Autodesk Inventor part; units mm, degrees
(part 2 of 2)
sketch "Sketch2" plane through (-23.7091, -13.8536, 14.2492) normal (0, 0.9970894, 0.0762418) x (1, 0, 0)
  line L0 (0.0409, 0.625) -> (-23.5591, 0.625) projected
  line L1 (0.0409, 0.625) -> (-23.5591, 0.625)
  line L2 (-23.5591, 0.625) -> (-23.5591, 65.9208)
  line L3 (-23.5591, 65.9208) -> (0.0409, 65.9208)
  line L4 (0.0409, 65.9208) -> (0.0409, 0.625)
  circle A0 centre (-9.1675, 23.6102) radius 8 construction
  circle A1 centre (-12.9591, 35.6262) radius 9.6 construction
  circle A2 centre (-9.1675, 23.6102) radius 8.4
  circle A3 centre (-12.9591, 35.6262) radius 10
  circle A4 centre (-9.1675, 23.6102) radius 1.25 projected
  arc A5 (-17.1384, 22.9282) -> (-15.9774, 22.6664) centre (-15.4653, 27.6426) ccw projected
  arc A6 (-15.9774, 22.6664) -> (-15.9187, 22.3113) centre (-9.1675, 23.6102) ccw projected
  arc A7 (-15.9187, 22.3113) -> (-16.9336, 21.6897) centre (-13.8318, 17.7649) ccw projected
  arc A8 (-16.9336, 21.6897) -> (-16.8224, 21.2858) centre (-9.1675, 23.6102) ccw projected
  arc A9 (-16.8224, 21.2858) -> (-15.6324, 21.2712) centre (-16.1661, 26.2451) ccw projected
  arc A10 (-15.6324, 21.2712) -> (-15.5011, 20.936) centre (-9.1675, 23.6102) ccw projected
  arc A11 (-15.5011, 20.936) -> (-16.3646, 20.117) centre (-12.5145, 16.9228) ccw projected
  arc A12 (-16.3646, 20.117) -> (-16.1719, 19.7451) centre (-9.1675, 23.6102) ccw projected
  arc A13 (-16.1719, 19.7451) -> (-15.0048, 19.9781) centre (-16.561, 24.7325) ccw projected
  arc A14 (-15.0048, 19.9781) -> (-14.8067, 19.6776) centre (-9.1675, 23.6102) ccw projected
  arc A15 (-14.8067, 19.6776) -> (-15.481, 18.697) centre (-11.051, 16.3731) ccw projected
  arc A16 (-15.481, 18.697) -> (-15.2152, 18.3733) centre (-9.1675, 23.6102) ccw projected
  arc A17 (-15.2152, 18.3733) -> (-14.1221, 18.8439) centre (-16.6328, 23.1708) ccw projected
  arc A18 (-14.1221, 18.8439) -> (-13.8659, 18.5911) centre (-9.1675, 23.6102) ccw projected
  arc A19 (-13.8659, 18.5911) -> (-14.3215, 17.4917) centre (-9.5052, 16.1397) ccw projected
  arc A20 (-14.3215, 17.4917) -> (-13.9942, 17.2303) centre (-9.1675, 23.6102) ccw projected
  arc A21 (-13.9942, 17.2303) -> (-13.0229, 17.9179) centre (-16.3783, 21.6283) ccw projected
  arc A22 (-13.0229, 17.9179) -> (-12.7197, 17.7239) centre (-9.1675, 23.6102) ccw projected
  arc A23 (-12.7197, 17.7239) -> (-12.9368, 16.5538) centre (-7.9446, 16.2327) ccw projected
  arc A24 (-12.9368, 16.5538) -> (-12.5623, 16.3662) centre (-9.1675, 23.6102) ccw projected
  arc A25 (-12.5623, 16.3662) -> (-11.7551, 17.2407) centre (-15.8086, 20.1724) ccw projected
  arc A26 (-11.7551, 17.2407) -> (-11.4182, 17.114) centre (-9.1675, 23.6102) ccw projected
  arc A27 (-11.4182, 17.114) -> (-11.3873, 15.9243) centre (-6.4374, 16.6482) ccw projected
  arc A28 (-11.3873, 15.9243) -> (-10.982, 15.8187) centre (-9.1675, 23.6102) ccw projected
  arc A29 (-10.982, 15.8187) -> (-10.3743, 16.8419) centre (-14.9487, 18.8667) ccw projected
  arc A30 (-10.3743, 16.8419) -> (-10.0184, 16.7881) centre (-9.1675, 23.6102) ccw projected
  arc A31 (-10.0184, 16.7881) -> (-9.7408, 15.6308) centre (-5.0496, 17.3679) ccw projected
  arc A32 (-9.7408, 15.6308) -> (-9.3224, 15.6117) centre (-9.1675, 23.6102) ccw projected
  arc A33 (-9.3224, 15.6117) -> (-8.9407, 16.7389) centre (-13.8362, 17.7684) ccw projected
  arc A34 (-8.9407, 16.7389) -> (-8.5814, 16.7602) centre (-9.1675, 23.6102) ccw projected
  arc A35 (-8.5814, 16.7602) -> (-8.0693, 15.6859) centre (-3.8418, 18.3605) ccw projected
  arc A36 (-8.0693, 15.6859) -> (-7.6561, 15.7543) centre (-9.1675, 23.6102) ccw projected
  arc A37 (-7.6561, 15.7543) -> (-7.5171, 16.9362) centre (-12.5196, 16.9254) ccw projected
  arc A38 (-7.5171, 16.9362) -> (-7.17, 17.0318) centre (-9.1675, 23.6102) ccw projected
  arc A39 (-7.17, 17.0318) -> (-6.4457, 16.0874) centre (-2.8667, 19.5825) ccw projected
  arc A40 (-6.4457, 16.0874) -> (-6.0558, 16.2402) centre (-9.1675, 23.6102) ccw projected
  arc A41 (-6.0558, 16.2402) -> (-6.1655, 17.4252) centre (-11.0565, 16.3745) ccw projected
  arc A42 (-6.1655, 17.4252) -> (-5.846, 17.5908) centre (-9.1675, 23.6102) ccw projected
  arc A43 (-5.846, 17.5908) -> (-4.9411, 16.8177) centre (-2.167, 20.9806) ccw projected
  arc A44 (-4.9411, 16.8177) -> (-4.5914, 17.0482) centre (-9.1675, 23.6102) ccw projected
  arc A45 (-4.5914, 17.0482) -> (-4.9452, 18.1845) centre (-9.5108, 16.1399) ccw projected
  arc A46 (-4.9452, 18.1845) -> (-4.667, 18.413) centre (-9.1675, 23.6102) ccw projected
  arc A47 (-4.667, 18.413) -> (-3.6213, 17.8449) centre (-1.7732, 22.4935) ccw projected
  arc A48 (-3.6213, 17.8449) -> (-3.3271, 18.143) centre (-9.1675, 23.6102) ccw projected
  arc A49 (-3.3271, 18.143) -> (-3.9094, 19.181) centre (-7.9502, 16.2318) ccw projected
  arc A50 (-3.9094, 19.181) -> (-3.6848, 19.4622) centre (-9.1675, 23.6102) ccw projected
  arc A51 (-3.6848, 19.4622) -> (-2.5438, 19.124) centre (-1.7026, 24.0553) ccw projected
  arc A52 (-2.5438, 19.124) -> (-2.3181, 19.4768) centre (-9.1675, 23.6102) ccw projected
  arc A53 (-2.3181, 19.4768) -> (-3.1034, 20.371) centre (-6.4427, 16.6461) ccw projected
  arc A54 (-3.1034, 20.371) -> (-2.9422, 20.6928) centre (-9.1675, 23.6102) ccw projected
  arc A55 (-2.9422, 20.6928) -> (-1.7558, 20.5992) centre (-1.9583, 25.5976) ccw projected
  arc A56 (-1.7558, 20.5992) -> (-1.6084, 20.9912) centre (-9.1675, 23.6102) ccw projected
  arc A57 (-1.6084, 20.9912) -> (-2.5625, 21.7026) centre (-5.0543, 17.3648) ccw projected
  arc A58 (-2.5625, 21.7026) -> (-2.4717, 22.0509) centre (-9.1675, 23.6102) ccw projected
  arc A59 (-2.4717, 22.0509) -> (-1.2917, 22.206) centre (-2.529, 27.0531) ccw projected
  arc A60 (-1.2917, 22.206) -> (-1.229, 22.6201) centre (-9.1675, 23.6102) ccw projected
  arc A61 (-1.229, 22.6201) -> (-2.3102, 23.1175) centre (-3.8457, 18.3565) ccw projected
  arc A62 (-2.3102, 23.1175) -> (-2.2938, 23.4771) centre (-9.1675, 23.6102) ccw projected
  arc A63 (-2.2938, 23.4771) -> (-1.1719, 23.8741) centre (-3.3899, 28.3581) ccw projected
  arc A64 (-1.1719, 23.8741) -> (-1.1967, 24.2922) centre (-9.1675, 23.6102) ccw projected
  arc A65 (-1.1967, 24.2922) -> (-2.3576, 24.554) centre (-2.8697, 19.5777) ccw projected
  arc A66 (-2.3576, 24.554) -> (-2.4163, 24.9091) centre (-9.1675, 23.6102) ccw projected
  arc A67 (-2.4163, 24.9091) -> (-1.4015, 25.5307) centre (-4.5033, 29.4555) ccw projected
  arc A68 (-1.4015, 25.5307) -> (-1.5126, 25.9345) centre (-9.1675, 23.6102) ccw projected
  arc A69 (-1.5126, 25.9345) -> (-2.7027, 25.9492) centre (-2.169, 20.9752) ccw projected
  arc A70 (-2.7027, 25.9492) -> (-2.8339, 26.2844) centre (-9.1675, 23.6102) ccw projected
  arc A71 (-2.8339, 26.2844) -> (-1.9705, 27.1034) centre (-5.8205, 30.2975) ccw projected
  arc A72 (-1.9705, 27.1034) -> (-2.1632, 27.4753) centre (-9.1675, 23.6102) ccw projected
  arc A73 (-2.1632, 27.4753) -> (-3.3302, 27.2422) centre (-1.7741, 22.4879) ccw projected
  arc A74 (-3.3302, 27.2422) -> (-3.5283, 27.5428) centre (-9.1675, 23.6102) ccw projected
  arc A75 (-3.5283, 27.5428) -> (-2.854, 28.5234) centre (-7.2841, 30.8473) ccw projected
  arc A76 (-2.854, 28.5234) -> (-3.1198, 28.8471) centre (-9.1675, 23.6102) ccw projected
  arc A77 (-3.1198, 28.8471) -> (-4.213, 28.3765) centre (-1.7023, 24.0496) ccw projected
  arc A78 (-4.213, 28.3765) -> (-4.4692, 28.6293) centre (-9.1675, 23.6102) ccw projected
  arc A79 (-4.4692, 28.6293) -> (-4.0135, 29.7287) centre (-8.8299, 31.0807) ccw projected
  arc A80 (-4.0135, 29.7287) -> (-4.3408, 29.9901) centre (-9.1675, 23.6102) ccw projected
  arc A81 (-4.3408, 29.9901) -> (-5.3122, 29.3025) centre (-1.9568, 25.5921) ccw projected
  arc A82 (-5.3122, 29.3025) -> (-5.6154, 29.4964) centre (-9.1675, 23.6102) ccw projected
  arc A83 (-5.6154, 29.4964) -> (-5.3983, 30.6666) centre (-10.3905, 30.9877) ccw projected
  arc A84 (-5.3983, 30.6666) -> (-5.7727, 30.8542) centre (-9.1675, 23.6102) ccw projected
  arc A85 (-5.7727, 30.8542) -> (-6.5799, 29.9797) centre (-2.5264, 27.048) ccw projected
  arc A86 (-6.5799, 29.9797) -> (-6.9168, 30.1063) centre (-9.1675, 23.6102) ccw projected
  arc A87 (-6.9168, 30.1063) -> (-6.9477, 31.2961) centre (-11.8976, 30.5722) ccw projected
  arc A88 (-6.9477, 31.2961) -> (-7.353, 31.4017) centre (-9.1675, 23.6102) ccw projected
  arc A89 (-7.353, 31.4017) -> (-7.9608, 30.3785) centre (-3.3863, 28.3537) ccw projected
  arc A90 (-7.9608, 30.3785) -> (-8.3166, 30.4323) centre (-9.1675, 23.6102) ccw projected
  arc A91 (-8.3166, 30.4323) -> (-8.5942, 31.5896) centre (-13.2855, 29.8524) ccw projected
  arc A92 (-8.5942, 31.5896) -> (-9.0126, 31.6087) centre (-9.1675, 23.6102) ccw projected
  arc A93 (-9.0126, 31.6087) -> (-9.3943, 30.4815) centre (-4.4989, 29.452) ccw projected
  arc A94 (-9.3943, 30.4815) -> (-9.7536, 30.4602) centre (-9.1675, 23.6102) ccw projected
  arc A95 (-9.7536, 30.4602) -> (-10.2658, 31.5345) centre (-14.4933, 28.8599) ccw projected
  arc A96 (-10.2658, 31.5345) -> (-10.679, 31.4661) centre (-9.1675, 23.6102) ccw projected
  arc A97 (-10.679, 31.4661) -> (-10.818, 30.2841) centre (-5.8155, 30.295) ccw projected
  arc A98 (-10.818, 30.2841) -> (-11.165, 30.1886) centre (-9.1675, 23.6102) ccw projected
  arc A99 (-11.165, 30.1886) -> (-11.8893, 31.1329) centre (-15.4684, 27.6379) ccw projected
  arc A100 (-11.8893, 31.1329) -> (-12.2793, 30.9802) centre (-9.1675, 23.6102) ccw projected
  arc A101 (-12.2793, 30.9802) -> (-12.1695, 29.7952) centre (-7.2786, 30.8459) ccw projected
  arc A102 (-12.1695, 29.7952) -> (-12.4891, 29.6296) centre (-9.1675, 23.6102) ccw projected
  arc A103 (-12.4891, 29.6296) -> (-13.3939, 30.4027) centre (-16.1681, 26.2398) ccw projected
  arc A104 (-13.3939, 30.4027) -> (-13.7436, 30.1722) centre (-9.1675, 23.6102) ccw projected
  arc A105 (-13.7436, 30.1722) -> (-13.3898, 29.0358) centre (-8.8242, 31.0805) ccw projected
  arc A106 (-13.3898, 29.0358) -> (-13.668, 28.8074) centre (-9.1675, 23.6102) ccw projected
  arc A107 (-13.668, 28.8074) -> (-14.7138, 29.3755) centre (-16.5619, 24.7269) ccw projected
  arc A108 (-14.7138, 29.3755) -> (-15.0079, 29.0774) centre (-9.1675, 23.6102) ccw projected
  arc A109 (-15.0079, 29.0774) -> (-14.4256, 28.0394) centre (-10.3849, 30.9886) ccw projected
  arc A110 (-14.4256, 28.0394) -> (-14.6502, 27.7582) centre (-9.1675, 23.6102) ccw projected
  arc A111 (-14.6502, 27.7582) -> (-15.7913, 28.0964) centre (-16.6324, 23.1651) ccw projected
  arc A112 (-15.7913, 28.0964) -> (-16.017, 27.7436) centre (-9.1675, 23.6102) ccw projected
  arc A113 (-16.017, 27.7436) -> (-15.2316, 26.8494) centre (-11.8923, 30.5743) ccw projected
  arc A114 (-15.2316, 26.8494) -> (-15.3928, 26.5276) centre (-9.1675, 23.6102) ccw projected
  arc A115 (-15.3928, 26.5276) -> (-16.5793, 26.6212) centre (-16.3768, 21.6228) ccw projected
  arc A116 (-16.5793, 26.6212) -> (-16.7267, 26.2292) centre (-9.1675, 23.6102) ccw projected
  arc A117 (-16.7267, 26.2292) -> (-15.7726, 25.5178) centre (-13.2807, 29.8556) ccw projected
  arc A118 (-15.7726, 25.5178) -> (-15.8634, 25.1695) centre (-9.1675, 23.6102) ccw projected
  arc A119 (-15.8634, 25.1695) -> (-17.0433, 25.0144) centre (-15.806, 20.1673) ccw projected
  arc A120 (-17.0433, 25.0144) -> (-17.106, 24.6003) centre (-9.1675, 23.6102) ccw projected
  arc A121 (-17.106, 24.6003) -> (-16.0249, 24.1029) centre (-14.4893, 28.8639) ccw projected
  arc A122 (-16.0249, 24.1029) -> (-16.0412, 23.7433) centre (-9.1675, 23.6102) ccw projected
  arc A123 (-16.0412, 23.7433) -> (-17.1632, 23.3463) centre (-14.9451, 18.8623) ccw projected
  arc A124 (-17.1632, 23.3463) -> (-17.1384, 22.9282) centre (-9.1675, 23.6102) ccw projected
  arc A125 (-20.5914, 38.7585) -> (-22.0189, 38.8013) centre (-21.4836, 32.8221) ccw projected
  arc A126 (-22.0189, 38.8013) -> (-22.1726, 38.3228) centre (-12.9591, 35.6262) ccw projected
  arc A127 (-22.1726, 38.3228) -> (-20.9874, 37.526) centre (-18.2546, 42.8709) ccw projected
  arc A128 (-20.9874, 37.526) -> (-21.0758, 37.1032) centre (-12.9591, 35.6262) ccw projected
  arc A129 (-21.0758, 37.1032) -> (-22.481, 36.8482) centre (-20.7143, 31.1111) ccw projected
  arc A130 (-22.481, 36.8482) -> (-22.5319, 36.3482) centre (-12.9591, 35.6262) ccw projected
  arc A131 (-22.5319, 36.3482) -> (-21.207, 35.8153) centre (-19.6452, 41.6116) ccw projected
  arc A132 (-21.207, 35.8153) -> (-21.2056, 35.3834) centre (-12.9591, 35.6262) ccw projected
  arc A133 (-21.2056, 35.3834) -> (-22.527, 34.8418) centre (-19.6061, 29.5973) ccw projected
  arc A134 (-22.527, 34.8418) -> (-22.4729, 34.3422) centre (-12.9591, 35.6262) ccw projected
  arc A135 (-22.4729, 34.3422) -> (-21.066, 34.0963) centre (-20.7435, 40.0907) ccw projected
  arc A136 (-21.066, 34.0963) -> (-20.9749, 33.6742) centre (-12.9591, 35.6262) ccw projected
  arc A137 (-20.9749, 33.6742) -> (-22.1549, 32.8697) centre (-18.2074, 28.3471) ccw projected
  arc A138 (-22.1549, 32.8697) -> (-21.998, 32.3922) centre (-12.9591, 35.6262) ccw projected
  arc A139 (-21.998, 32.3922) -> (-20.5708, 32.4442) centre (-21.5017, 38.3747) ccw projected
  arc A140 (-20.5708, 32.4442) -> (-20.3939, 32.0502) centre (-12.9591, 35.6262) ccw projected
  arc A141 (-20.3939, 32.0502) -> (-21.3808, 31.018) centre (-16.5793, 27.415) ccw projected
  arc A142 (-21.3808, 31.018) -> (-21.1281, 30.5836) centre (-12.9591, 35.6262) ccw projected
  arc A143 (-21.1281, 30.5836) -> (-19.7429, 30.9312) centre (-21.8864, 36.5385) ccw projected
  arc A144 (-19.7429, 30.9312) -> (-19.4879, 30.5826) centre (-12.9591, 35.6262) ccw projected
  arc A145 (-19.4879, 30.5826) -> (-20.2387, 29.3677) centre (-14.793, 26.8417) ccw projected
  arc A146 (-20.2387, 29.3677) -> (-19.9012, 28.9953) centre (-12.9591, 35.6262) ccw projected
  arc A147 (-19.9012, 28.9953) -> (-18.6186, 29.6234) centre (-21.881, 34.6625) ccw projected
  arc A148 (-18.6186, 29.6234) -> (-18.2966, 29.3354) centre (-12.9591, 35.6262) ccw projected
  arc A149 (-18.2966, 29.3354) -> (-18.7784, 27.991) centre (-12.9265, 26.6524) ccw projected
  arc A150 (-18.7784, 27.991) -> (-18.3709, 27.6969) centre (-12.9591, 35.6262) ccw projected
  arc A151 (-18.3709, 27.6969) -> (-17.2468, 28.5779) centre (-21.4857, 32.8286) ccw projected
  arc A152 (-17.2468, 28.5779) -> (-16.8721, 28.3632) centre (-12.9591, 35.6262) ccw projected
  arc A153 (-16.8721, 28.3632) -> (-17.0638, 26.948) centre (-11.0615, 26.8553) ccw projected
  arc A154 (-17.0638, 26.948) -> (-16.604, 26.745) centre (-12.9591, 35.6262) ccw projected
  arc A155 (-16.604, 26.745) -> (-15.6877, 27.8405) centre (-20.7177, 31.117) ccw projected
  arc A156 (-15.6877, 27.8405) -> (-15.2765, 27.7083) centre (-12.9591, 35.6262) ccw projected
  arc A157 (-15.2765, 27.7083) -> (-15.1698, 26.2842) centre (-9.2794, 27.4415) ccw projected
  arc A158 (-15.1698, 26.2842) -> (-14.6779, 26.1813) centre (-12.9591, 35.6262) ccw projected
  arc A159 (-14.6779, 26.1813) -> (-14.0093, 27.4433) centre (-19.6107, 29.6024) ccw projected
  arc A160 (-14.0093, 27.4433) -> (-13.5796, 27.3995) centre (-12.9591, 35.6262) ccw projected
  arc A161 (-13.5796, 27.3995) -> (-13.1792, 26.0287) centre (-7.6581, 28.3854) ccw projected
  arc A162 (-13.1792, 26.0287) -> (-12.6766, 26.0303) centre (-12.9591, 35.6262) ccw projected
  arc A163 (-12.6766, 26.0303) -> (-12.2851, 27.4038) centre (-18.2129, 28.3511) ccw projected
  arc A164 (-12.2851, 27.4038) -> (-11.8557, 27.4503) centre (-12.9591, 35.6262) ccw projected
  arc A165 (-11.8557, 27.4503) -> (-11.179, 26.1927) centre (-6.2685, 29.6458) ccw projected
  arc A166 (-11.179, 26.1927) -> (-10.6877, 26.2988) centre (-12.9591, 35.6262) ccw projected
  arc A167 (-10.6877, 26.2988) -> (-10.5903, 27.7236) centre (-16.5855, 27.4177) ccw projected
  arc A168 (-10.5903, 27.7236) -> (-10.1799, 27.8584) centre (-12.9591, 35.6262) ccw projected
  arc A169 (-10.1799, 27.8584) -> (-9.2565, 26.7689) centre (-5.1713, 31.1675) ccw projected
  arc A170 (-9.2565, 26.7689) -> (-8.798, 26.9749) centre (-12.9591, 35.6262) ccw projected
  arc A171 (-8.798, 26.9749) -> (-8.999, 28.3888) centre (-14.7996, 26.8431) ccw projected
  arc A172 (-8.999, 28.3888) -> (-8.6256, 28.606) centre (-12.9591, 35.6262) ccw projected
  arc A173 (-8.6256, 28.606) -> (-7.4959, 27.7323) centre (-4.4145, 32.8842) ccw projected
  arc A174 (-7.4959, 27.7323) -> (-7.0903, 28.029) centre (-12.9591, 35.6262) ccw projected
  arc A175 (-7.0903, 28.029) -> (-7.5808, 29.3703) centre (-12.9333, 26.6524) ccw projected
  arc A176 (-7.5808, 29.3703) -> (-7.2608, 29.6603) centre (-12.9591, 35.6262) ccw projected
  arc A177 (-7.2608, 29.6603) -> (-5.9741, 29.0407) centre (-4.0311, 34.7206) ccw projected
  arc A178 (-5.9741, 29.0407) -> (-5.639, 29.4153) centre (-12.9591, 35.6262) ccw projected
  arc A179 (-5.639, 29.4153) -> (-6.3977, 30.6252) centre (-11.0681, 26.8539) ccw projected
  arc A180 (-6.3977, 30.6252) -> (-6.1449, 30.9755) centre (-12.9591, 35.6262) ccw projected
  arc A181 (-6.1449, 30.9755) -> (-4.7575, 30.6369) centre (-4.038, 36.5966) ccw projected
  arc A182 (-4.7575, 30.6369) -> (-4.5076, 31.0729) centre (-12.9591, 35.6262) ccw projected
  arc A183 (-4.5076, 31.0729) -> (-5.5013, 32.0987) centre (-9.2856, 27.4387) ccw projected
  arc A184 (-5.5013, 32.0987) -> (-5.3269, 32.4939) centre (-12.9591, 35.6262) ccw projected
  arc A185 (-5.3269, 32.4939) -> (-3.8994, 32.4511) centre (-4.4347, 38.4302) ccw projected
  arc A186 (-3.8994, 32.4511) -> (-3.7456, 32.9296) centre (-12.9591, 35.6262) ccw projected
  arc A187 (-3.7456, 32.9296) -> (-4.9309, 33.7264) centre (-7.6636, 28.3814) ccw projected
  arc A188 (-4.9309, 33.7264) -> (-4.8424, 34.1491) centre (-12.9591, 35.6262) ccw projected
  arc A189 (-4.8424, 34.1491) -> (-3.4372, 34.4041) centre (-5.2039, 40.1413) ccw projected
  arc A190 (-3.4372, 34.4041) -> (-3.3863, 34.9041) centre (-12.9591, 35.6262) ccw projected
  arc A191 (-3.3863, 34.9041) -> (-4.7113, 35.4371) centre (-6.2731, 29.6407) ccw projected
  arc A192 (-4.7113, 35.4371) -> (-4.7127, 35.869) centre (-12.9591, 35.6262) ccw projected
  arc A193 (-4.7127, 35.869) -> (-3.3912, 36.4105) centre (-6.3122, 41.655) ccw projected
  arc A194 (-3.3912, 36.4105) -> (-3.4454, 36.9102) centre (-12.9591, 35.6262) ccw projected
  arc A195 (-3.4454, 36.9102) -> (-4.8522, 37.156) centre (-5.1747, 31.1616) ccw projected
  arc A196 (-4.8522, 37.156) -> (-4.9434, 37.5782) centre (-12.9591, 35.6262) ccw projected
  arc A197 (-4.9434, 37.5782) -> (-3.7634, 38.3827) centre (-7.7109, 42.9053) ccw projected
  arc A198 (-3.7634, 38.3827) -> (-3.9202, 38.8602) centre (-12.9591, 35.6262) ccw projected
  arc A199 (-3.9202, 38.8602) -> (-5.3474, 38.8081) centre (-4.4166, 32.8777) ccw projected
  arc A200 (-5.3474, 38.8081) -> (-5.5244, 39.2021) centre (-12.9591, 35.6262) ccw projected
  arc A201 (-5.5244, 39.2021) -> (-4.5374, 40.2343) centre (-9.339, 43.8374) ccw projected
  arc A202 (-4.5374, 40.2343) -> (-4.7902, 40.6688) centre (-12.9591, 35.6262) ccw projected
  arc A203 (-4.7902, 40.6688) -> (-6.1753, 40.3211) centre (-4.0318, 34.7138) ccw projected
  arc A204 (-6.1753, 40.3211) -> (-6.4303, 40.6697) centre (-12.9591, 35.6262) ccw projected
  arc A205 (-6.4303, 40.6697) -> (-5.6796, 41.8846) centre (-11.1253, 44.4106) ccw projected
  arc A206 (-5.6796, 41.8846) -> (-6.0171, 42.257) centre (-12.9591, 35.6262) ccw projected
  arc A207 (-6.0171, 42.257) -> (-7.2997, 41.629) centre (-4.0372, 36.5898) ccw projected
  arc A208 (-7.2997, 41.629) -> (-7.6216, 41.9169) centre (-12.9591, 35.6262) ccw projected
  arc A209 (-7.6216, 41.9169) -> (-7.1398, 43.2613) centre (-12.9917, 44.5999) ccw projected
  arc A210 (-7.1398, 43.2613) -> (-7.5474, 43.5554) centre (-12.9591, 35.6262) ccw projected
  arc A211 (-7.5474, 43.5554) -> (-8.6714, 42.6744) centre (-4.4325, 38.4238) ccw projected
  arc A212 (-8.6714, 42.6744) -> (-9.0462, 42.8892) centre (-12.9591, 35.6262) ccw projected
  arc A213 (-9.0462, 42.8892) -> (-8.8544, 44.3044) centre (-14.8568, 44.397) ccw projected
  arc A214 (-8.8544, 44.3044) -> (-9.3143, 44.5073) centre (-12.9591, 35.6262) ccw projected
  arc A215 (-9.3143, 44.5073) -> (-10.2305, 43.4119) centre (-5.2005, 40.1354) ccw projected
  arc A216 (-10.2305, 43.4119) -> (-10.6418, 43.544) centre (-12.9591, 35.6262) ccw projected
  arc A217 (-10.6418, 43.544) -> (-10.7484, 44.9682) centre (-16.6389, 43.8108) ccw projected
  arc A218 (-10.7484, 44.9682) -> (-11.2404, 45.0711) centre (-12.9591, 35.6262) ccw projected
  arc A219 (-11.2404, 45.0711) -> (-11.9089, 43.8091) centre (-6.3076, 41.65) ccw projected
  arc A220 (-11.9089, 43.8091) -> (-12.3386, 43.8528) centre (-12.9591, 35.6262) ccw projected
  arc A221 (-12.3386, 43.8528) -> (-12.7391, 45.2237) centre (-18.2601, 42.8669) ccw projected
  arc A222 (-12.7391, 45.2237) -> (-13.2417, 45.222) centre (-12.9591, 35.6262) ccw projected
  arc A223 (-13.2417, 45.222) -> (-13.6332, 43.8486) centre (-7.7054, 42.9013) ccw projected
  arc A224 (-13.6332, 43.8486) -> (-14.0626, 43.802) centre (-12.9591, 35.6262) ccw projected
  arc A225 (-14.0626, 43.802) -> (-14.7393, 45.0597) centre (-19.6497, 41.6065) ccw projected
  arc A226 (-14.7393, 45.0597) -> (-15.2306, 44.9536) centre (-12.9591, 35.6262) ccw projected
  arc A227 (-15.2306, 44.9536) -> (-15.328, 43.5288) centre (-9.3327, 43.8346) ccw projected
  arc A228 (-15.328, 43.5288) -> (-15.7383, 43.394) centre (-12.9591, 35.6262) ccw projected
  arc A229 (-15.7383, 43.394) -> (-16.6617, 44.4834) centre (-20.7469, 40.0848) ccw projected
  arc A230 (-16.6617, 44.4834) -> (-17.1202, 44.2775) centre (-12.9591, 35.6262) ccw projected
  arc A231 (-17.1202, 44.2775) -> (-16.9193, 42.8636) centre (-11.1186, 44.4092) ccw projected
  arc A232 (-16.9193, 42.8636) -> (-17.2926, 42.6464) centre (-12.9591, 35.6262) ccw projected
  arc A233 (-17.2926, 42.6464) -> (-18.4223, 43.52) centre (-21.5037, 38.3682) ccw projected
  arc A234 (-18.4223, 43.52) -> (-18.828, 43.2233) centre (-12.9591, 35.6262) ccw projected
  arc A235 (-18.828, 43.2233) -> (-18.3375, 41.8821) centre (-12.9849, 44.5999) ccw projected
  arc A236 (-18.3375, 41.8821) -> (-18.6575, 41.592) centre (-12.9591, 35.6262) ccw projected
  arc A237 (-18.6575, 41.592) -> (-19.9442, 42.2117) centre (-21.8871, 36.5318) ccw projected
  arc A238 (-19.9442, 42.2117) -> (-20.2793, 41.8371) centre (-12.9591, 35.6262) ccw projected
  arc A239 (-20.2793, 41.8371) -> (-19.5206, 40.6271) centre (-14.8501, 44.3985) ccw projected
  arc A240 (-19.5206, 40.6271) -> (-19.7733, 40.2769) centre (-12.9591, 35.6262) ccw projected
  arc A241 (-19.7733, 40.2769) -> (-21.1608, 40.6155) centre (-21.8803, 34.6557) ccw projected
  arc A242 (-21.1608, 40.6155) -> (-21.4106, 40.1794) centre (-12.9591, 35.6262) ccw projected
  arc A243 (-21.4106, 40.1794) -> (-20.417, 39.1536) centre (-16.6327, 43.8136) ccw projected
  arc A244 (-20.417, 39.1536) -> (-20.5914, 38.7585) centre (-12.9591, 35.6262) ccw projected
  circle A245 centre (-14.4591, 55.9208) radius 14.5 projected
  circle A246 centre (-14.4591, 55.9208) radius 13.85 projected
  circle A247 centre (-14.4591, 15.125) radius 14.5 projected
  circle A248 centre (-14.4591, 15.125) radius 13.85 projected
  circle A249 centre (-14.4591, 15.125) radius 5 projected
  circle A250 centre (-12.9591, 35.6262) radius 5 projected
  point P0 (23.7091, 15.264)
  point P1 (-7.7492, 27.5629)
  point P2 (-4.3698, 30.5053)
  point P3 (-17.0537, 26.5029)
  point P4 (-23.5591, 0.625)
  point P5 (-5.7766, 30.8509)
  point P6 (-5.7466, 30.8419)
  point P7 (-15.2552, 26.8707)
  point P8 (-15.2497, 26.8153)
  point P9 (-9.4599, 15.2153)
  point P10 (-16.5776, 19.654)
  dimension "d14" = 0.4
  dimension "d15" = 0.4
  dimension "d16" = 0.6
  dimension "d140" = 4.5
  constraints: 8 end point, 3 centre point, 2 coincident, 2 parallel, 2 point on circle, 1 horizontal, 1 perpendicular, 4 other
  measures "d15" radial gap between concentric circles of A1 A3
  measures "d16" distance edge to line of A3 L2
  measures "d140" distance edge to line of A245 L3
extrude "Extrusion5" add sketch "Sketch2" along normal blind 3.7 contours L0 A247 L4 | L0 L2 A247 | A247 L2 A248 A2 | A247 A2 A3 A245 L4 | A245 L3 L4 | A245 A3 A246 L3 | L2 A248 A3 A2 A249 | A247 A3 A248 L2 | L2 A245 A3 A247 | L2 A246 A3 A245 | A246 A3 L2 L3
ref_plane "Work Plane7" through (-38.1326, -18.2417, -0.502) normal (0, 0.9970894, 0.0762418) x (-0.6440904, -0.0583212, 0.7627229)
sketch "Sketch12" plane through (-38.1326, -18.2417, -0.502) normal (0, 0.9970894, 0.0762418) x (-0.6440904, -0.0583212, 0.7627229)
  circle A0 centre (-10.4391, -1.9494) radius 4.2 construction
  circle A1 centre (-10.4391, -1.9494) radius 4.6
  circle A2 centre (-10.4391, -1.9494) radius 1.25 projected
  arc A3 (-14.2545, -0.1936) -> (-13.1615, -1.1061) centre (-11.3781, 2.141) ccw projected
  arc A4 (-13.1615, -1.1061) -> (-13.2483, -1.4686) centre (-10.4391, -1.9494) ccw projected
  arc A5 (-13.2483, -1.4686) -> (-14.636, -1.7873) centre (-13.1285, -5.1712) ccw projected
  arc A6 (-14.636, -1.7873) -> (-14.6212, -2.3365) centre (-10.4391, -1.9494) ccw projected
  arc A7 (-14.6212, -2.3365) -> (-13.2184, -2.5802) centre (-13.2974, 1.1235) ccw projected
  arc A8 (-13.2184, -2.5802) -> (-13.1123, -2.9376) centre (-10.4391, -1.9494) ccw projected
  arc A9 (-13.1123, -2.9376) -> (-14.1548, -3.9074) centre (-11.1572, -6.0843) ccw projected
  arc A10 (-14.1548, -3.9074) -> (-13.8674, -4.3757) centre (-10.4391, -1.9494) ccw projected
  arc A11 (-13.8674, -4.3757) -> (-12.5307, -3.8854) centre (-14.4509, -0.7174) ccw projected
  arc A12 (-12.5307, -3.8854) -> (-12.2601, -4.1418) centre (-10.4391, -1.9494) ccw projected
  arc A13 (-12.2601, -4.1418) -> (-12.6779, -5.5029) centre (-8.9936, -5.8894) ccw projected
  arc A14 (-12.6779, -5.5029) -> (-12.195, -5.7648) centre (-10.4391, -1.9494) ccw projected
  arc A15 (-12.195, -5.7648) -> (-11.2825, -4.6718) centre (-14.5295, -2.8884) ccw projected
  arc A16 (-11.2825, -4.6718) -> (-10.9199, -4.7586) centre (-10.4391, -1.9494) ccw projected
  arc A17 (-10.9199, -4.7586) -> (-10.6012, -6.1463) centre (-7.2173, -4.6388) ccw projected
  arc A18 (-10.6012, -6.1463) -> (-10.052, -6.1315) centre (-10.4391, -1.9494) ccw projected
  arc A19 (-10.052, -6.1315) -> (-9.8083, -4.7287) centre (-13.512, -4.8077) ccw projected
  arc A20 (-9.8083, -4.7287) -> (-9.4509, -4.6226) centre (-10.4391, -1.9494) ccw projected
  arc A21 (-9.4509, -4.6226) -> (-8.4811, -5.6651) centre (-6.3043, -2.6675) ccw projected
  arc A22 (-8.4811, -5.6651) -> (-8.0128, -5.3777) centre (-10.4391, -1.9494) ccw projected
  arc A23 (-8.0128, -5.3777) -> (-8.5032, -4.041) centre (-11.6711, -5.9612) ccw projected
  arc A24 (-8.5032, -4.041) -> (-8.2467, -3.7704) centre (-10.4391, -1.9494) ccw projected
  arc A25 (-8.2467, -3.7704) -> (-6.8856, -4.1882) centre (-6.4992, -0.5039) ccw projected
  arc A26 (-6.8856, -4.1882) -> (-6.6238, -3.7053) centre (-10.4391, -1.9494) ccw projected
  arc A27 (-6.6238, -3.7053) -> (-7.7167, -2.7928) centre (-9.5002, -6.0398) ccw projected
  arc A28 (-7.7167, -2.7928) -> (-7.63, -2.4302) centre (-10.4391, -1.9494) ccw projected
  arc A29 (-7.63, -2.4302) -> (-6.2422, -2.1115) centre (-7.7498, 1.2724) ccw projected
  arc A30 (-6.2422, -2.1115) -> (-6.257, -1.5623) centre (-10.4391, -1.9494) ccw projected
  arc A31 (-6.257, -1.5623) -> (-7.6598, -1.3186) centre (-7.5808, -5.0223) ccw projected
  arc A32 (-7.6598, -1.3186) -> (-7.7659, -0.9612) centre (-10.4391, -1.9494) ccw projected
  arc A33 (-7.7659, -0.9612) -> (-6.7235, 0.0086) centre (-9.721, 2.1854) ccw projected
  arc A34 (-6.7235, 0.0086) -> (-7.0108, 0.4769) centre (-10.4391, -1.9494) ccw projected
  arc A35 (-7.0108, 0.4769) -> (-8.3476, -0.0134) centre (-6.4273, -3.1814) ccw projected
  arc A36 (-8.3476, -0.0134) -> (-8.6182, 0.243) centre (-10.4391, -1.9494) ccw projected
  arc A37 (-8.6182, 0.243) -> (-8.2003, 1.6041) centre (-11.8846, 1.9905) ccw projected
  arc A38 (-8.2003, 1.6041) -> (-8.6833, 1.866) centre (-10.4391, -1.9494) ccw projected
  arc A39 (-8.6833, 1.866) -> (-9.5958, 0.773) centre (-6.3487, -1.0105) ccw projected
  arc A40 (-9.5958, 0.773) -> (-9.9583, 0.8597) centre (-10.4391, -1.9494) ccw projected
  arc A41 (-9.9583, 0.8597) -> (-10.277, 2.2475) centre (-13.6609, 0.7399) ccw projected
  arc A42 (-10.277, 2.2475) -> (-10.8262, 2.2327) centre (-10.4391, -1.9494) ccw projected
  arc A43 (-10.8262, 2.2327) -> (-11.0699, 0.8299) centre (-7.3662, 0.9089) ccw projected
  arc A44 (-11.0699, 0.8299) -> (-11.4273, 0.7238) centre (-10.4391, -1.9494) ccw projected
  arc A45 (-11.4273, 0.7238) -> (-12.3971, 1.7662) centre (-14.574, -1.2313) ccw projected
  arc A46 (-12.3971, 1.7662) -> (-12.8654, 1.4789) centre (-10.4391, -1.9494) ccw projected
  arc A47 (-12.8654, 1.4789) -> (-12.3751, 0.1421) centre (-9.2071, 2.0624) ccw projected
  arc A48 (-12.3751, 0.1421) -> (-12.6315, -0.1285) centre (-10.4391, -1.9494) ccw projected
  arc A49 (-12.6315, -0.1285) -> (-13.9926, 0.2894) centre (-14.3791, -3.3949) ccw projected
  arc A50 (-13.9926, 0.2894) -> (-14.2545, -0.1936) centre (-10.4391, -1.9494) ccw projected
  point P0 (-25.2418, 28.5962)
  point P1 (-6.3346, -1.0591)
  dimension "d110" = 0.4
  constraints: 2 centre point, 2 point on circle, 1 coincident
  measures "d110" radial gap between concentric circles of A0 A1
extrude "Extrusion9" add sketch "Sketch12" along normal blind 1.5 contours A1 | A2 | A50 A49 A48 A47 A46 A45 A44 A43 A42 A41 A40 A39 A38 A37 A36 A35 A34 A33 A32 A31 A30 A29 A28 A27 A26 A25 A24 A23 A22 A21 A20 A19 A18 A17 A16 A15 A14 A13 A12 A11 A10 A9 A8 A7 A6 A5 A4 A3
sketch "Sketch3" plane through (-23.7091, -10.1644, 14.5313) normal (0, 0.9970894, 0.0762418) x (1, 0, 0)
  line L0 (-1.5, 17.125) -> (-1.5, 1.125) projected
  line L1 (-2.5, 17.125) -> (-1.5, 17.125) projected
  line L2 (-2.5, 1.125) -> (-2.5, 17.125) projected
  line L3 (-2.5, 1.125) -> (-1.5, 1.125) projected
  line L4 (-1.5, 1.125) -> (-1, 1.125)
  line L5 (-1, 1.125) -> (-1, 17.625)
  line L6 (-1, 17.625) -> (-2.5, 17.625)
  line L7 (-2.5, 17.625) -> (-2.5, 17.125)
  point P0 (23.7091, 15.264)
  dimension "d20" = 0.5
  dimension "d21" = 0.5
  constraints: 8 end point, 3 perpendicular, 1 horizontal
  measures "d20" distance between parallel lines of L6 L1
  measures "d21" distance between parallel lines of L5 L0
extrude "Extrusion6" cut sketch "Sketch3" against normal blind 7.1
sketch "Sketch4" plane through (-23.7091, -10.1644, 14.5313) normal (0, 0.9970894, 0.0762418) x (1, 0, 0)
  line L0 (-1.4591, 17.125) -> (-1.4591, 1.125) projected
  line L1 (-2.4591, 17.125) -> (-1.4591, 17.125) projected
  line L2 (-2.4591, 1.125) -> (-2.4591, 17.125) projected
  line L3 (-2.5, 1.125) -> (-1.4591, 1.125) projected
  line L4 (-1.5, 4.225) -> (-1.5, 7.725) projected
  line L5 (-1.5, 4.225) -> (0, 4.225) projected
  line L6 (0, 7.725) -> (0, 4.225) projected
  line L7 (-1.5, 7.725) -> (0, 7.725) projected
  line L8 (-1.5, 10.525) -> (-1.5, 14.025) projected
  line L9 (-1.5, 10.525) -> (0, 10.525) projected
  line L10 (0, 14.025) -> (0, 10.525) projected
  line L11 (-1.5, 14.025) -> (0, 14.025) projected
  line L12 (0.5, 3.725) -> (-2, 3.725)
  line L13 (-2, 3.725) -> (-2, 8.225)
  line L14 (-2, 8.225) -> (0.5, 8.225)
  line L15 (0.5, 8.225) -> (0.5, 3.725)
  line L16 (0.5, 10.025) -> (-2, 10.025)
  line L17 (-2, 10.025) -> (-2, 14.525)
  line L18 (-2, 14.525) -> (0.5, 14.525)
  line L19 (0.5, 14.525) -> (0.5, 10.025)
  line L20 (-1, 1.125) -> (-2.5, 1.125) projected
  line L21 (-1.4591, 1.125) -> (-1, 1.125)
  line L22 (-1, 1.125) -> (-1, 17.625)
  line L23 (-1, 17.625) -> (-2.4591, 17.625)
  line L24 (-2.4591, 17.625) -> (-2.4591, 17.125)
  line L25 (-2.5, 1.125) -> (-2.5, 0.625)
  line L26 (0.0409, 0.625) -> (-23.5591, 0.625) projected
  line L27 (-2.5, 0.625) -> (0.0409, 0.625)
  line L28 (0.0409, 0.625) -> (0.0409, 16.9971)
  line L29 (0.0409, 65.9208) -> (0.0409, 0.625) projected
  line L30 (-2.4591, 17.625) -> (-2.4591, 18.625)
  line L31 (-2.4068, 18.625) -> (0.0409, 18.625)
  arc A0 (-9.4599, 15.2153) -> (-4.3698, 30.5053) centre (-9.1675, 23.6102) ccw projected
  point P0 (23.7091, 15.264)
  point P1 (-16.767, 19.3208)
  point P2 (0.0409, 3.725)
  point P3 (-1, 3.725)
  point P4 (0.0409, 8.225)
  point P5 (0.0409, 10.025)
  point P6 (-1, 10.025)
  point P7 (-1, 8.225)
  point P8 (-1, 14.525)
  point P9 (0.0409, 14.525)
  point P10 (-2.4591, 18.5548)
  point P11 (-15.0841, 28.9882)
  point P12 (-1.5756, 19.4781)
  point P13 (-1.1642, 20.5664)
  point P14 (0.0409, 14.525)
  point P15 (0.0409, 10.025)
  point P16 (-1.4591, 8.225)
  point P17 (-1.4591, 3.725)
  point P18 (-9.5166, 14.5909)
  point P19 (-9.5008, 15.2153)
  point P20 (-1.4591, 1.125)
  point P21 (0, 14.025)
  point P22 (0, 10.525)
  dimension "d24" = 0.5
  dimension "d25" = 0.5
  dimension "d26" = 0.5
  dimension "d27" = 1
  constraints: 34 end point, 3 perpendicular, 2 horizontal, 2 point on line, 2 vertical, 1 collinear, 1 point on circle, 11 other
  measures "d24" distance between parallel lines of L5 L12
  measures "d25" distance between parallel lines of L9 L16
  measures "d26" distance between parallel lines of L1 L23
  measures "d27" distance between parallel lines of L23 L31
extrude "Extrusion7" add sketch "Sketch4" along normal blind 8 contours L22 L23 L30 A0 L31 L29 L28 L18 | L3 L20 L22 L12 L28 L26 L25 | L0 L12 L22 L20
sketch "Sketch6" plane through (-23.7091, -10.1644, 14.5313) normal (0, 0.9970894, 0.0762418) x (1, 0, 0)
  circle A0 centre (-20.6284, 20.2673) radius 2.25 projected
  circle A1 centre (-8.3716, 9.9827) radius 2.25 projected
  point P0 (23.7091, 15.264)
extrude "Extrusion8" cut sketch "Sketch6" against normal blind 2.6
sketch "Sketch7" plane through (-44.3375, -11.2116, -5.8752) normal (0, 0.9970894, 0.0762418) x (1, 0, 0)
  circle A0 centre (0, 0) radius 2.25 projected
  circle A1 centre (12.2567, -10.2846) radius 2.25 projected
  point P0 (44.3375, -5.0033)
hole "Hole2" at (-44.3375, -11.2116, -5.8752) at (-32.0808, -11.9957, 4.3794) direction (0, -0.9970894, -0.0762418) diameter 2.5 depth 10.6 counterbore diameter 4.5 counterbore depth 2.6
sketch "Sketch5" plane through (-23.6683, -14.3117, -51.8991) normal (0, 0.0762418, -0.9970894) x (-1, 0, 0)
  line L0 (23.2, 5.4939) -> (6.7249, 5.4939)
  line L1 (6, 9.9939) -> (6, 1.4939)
  circle A0 centre (16.7, 7.3439) radius 3.5
  circle A1 centre (9.5, 7.3439) radius 3.5
  point P0 (-23.6683, 18.2269)
  point P1 (23.6, 9.2)
  point P2 (5.9014, 4.6)
  point P3 (6.7249, 5.4939)
  dimension "d49" = 7
  dimension "d50" = 7
  dimension "d51" = 1.85
  dimension "d53" = 1.85
  constraints: 2 centre point, 2 end point, 1 tangent, 3 other
  measures "d49" diameter of A0
  measures "d50" diameter of A1
hole "Hole1" at (-40.3683, -6.9892, -51.3392) at (-33.1683, -6.9892, -51.3392) direction (0, -0.0762418, 0.9970894) diameter 2.459 depth 5 countersink diameter 3 countersink angle 90 thread size "M3x0.5" class "6H" standard "ISO Metric profile"
sketch "Sketch9" plane through (-57.1953, -16.3972, -4.9503) normal (0, 0.9970894, 0.0762418) x (-0.1905215, -0.0748453, 0.9788257)
  arc A0 (-5.6026, 30.5719) -> (-16.8912, 26.3814) centre (-9.2084, 22.9852) ccw projected
  point P0 (-7.2787, 56.8498)
  point P1 (-2.4477, 18)
  point P2 (-1.5756, 19.4781)
  point P3 (-9.5008, 14.5903)
  point P4 (-17.2526, 25.404)
hole "Hole3" at (-32.8767, -16.0419, -9.5972) direction (0, -0.9970894, -0.0762418) diameter 2.5 depth 1.3
sketch "Sketch10" plane through (-23.7091, -10.1644, 14.5313) normal (0, 0.9970894, 0.0762418) x (1, 0, 0)
  line L0 (-23.5591, 65.9208) -> (-23.5591, 0.625) projected
  circle A0 centre (-3.4591, 61.7958) radius 3.5
  line L1 (0.0409, 0.625) -> (0.0409, 65.9208) projected
  circle A1 centre (-19.5591, 8.875) radius 3.5
  circle A2 centre (-20.0591, 47.5251) radius 3.5
  circle A3 centre (-3.3927, 45.0154) radius 3.5
  line L2 (-23.5591, 5.375) -> (-2.5, 5.375)
  line L3 (-0.9873, 13.625) -> (-23.5591, 13.625)
  circle A4 centre (-19.5591, 8.875) radius 2.5
  circle A5 centre (-19.9718, 24.9717) radius 3.5
  circle A6 centre (-19.9718, 24.9717) radius 2.5
  circle A7 centre (-20.6284, 20.2673) radius 2.25 projected
  line L4 (-23.5591, 0.625) -> (-2.5, 0.625) projected
  line L5 (0.0409, 65.9208) -> (-23.5591, 65.9208) projected
  line L6 (-2.5, 1.125) -> (-2.5, 17.625) projected
  line L7 (0.0409, 18.625) -> (0.0409, 65.9208) projected
  line L8 (0.0409, 14.525) -> (-1, 14.525) projected
  line L9 (-2.5, 0.625) -> (-2.5, 1.125) projected
  line L10 (-1, 3.725) -> (0.0409, 3.725) projected
  line L11 (0.0409, 3.725) -> (0.0409, 14.525) projected
  line L12 (-2.4068, 18.625) -> (0.0409, 18.625) projected
  line L13 (-2.4591, 17.625) -> (-2.4591, 18.5548) projected
  line L14 (-1, 14.525) -> (-1, 3.725) projected
  line L15 (-2.5, 17.625) -> (-2.4591, 17.625) projected
  arc A8 (-9.4599, 15.2153) -> (-2.4591, 18.5548) centre (-9.1675, 23.6102) ccw projected
  arc A9 (-16.5776, 19.654) -> (-9.4599, 15.2153) centre (-14.4591, 15.125) ccw projected
  arc A10 (-17.0537, 26.5029) -> (-16.5776, 19.654) centre (-9.1675, 23.6102) ccw projected
  arc A11 (-4.3698, 30.5053) -> (-17.0537, 26.5029) centre (-12.9591, 35.6262) ccw projected
  arc A12 (-2.4068, 18.625) -> (-4.3698, 30.5053) centre (-9.1675, 23.6102) ccw projected
  point P0 (23.7091, 15.264)
  dimension "d75" = 7
  dimension "d76" = 7
  dimension "d78" = 7
  dimension "d79" = 7
  dimension "d89" = 8.25
  dimension "d90" = 3.5
  dimension "d91" = 4.75
  dimension "d93" = 4
  dimension "d96" = 5
  dimension "d113" = 7
  dimension "d114" = 5
  dimension "d129" = 4.75
  constraints: 7 centre point, 4 end point, 3 tangent, 2 coincident, 2 point on line, 1 perpendicular
  measures "d75" diameter of A0
  measures "d76" diameter of A1
  measures "d78" diameter of A2
  measures "d79" diameter of A3
  measures "d89" distance between parallel lines of L3 L2
  measures "d90" distance from line of L2 A1.centre
  measures "d91" distance from line of L3 A1.centre
  measures "d93" distance from line of L0 A1.centre
  measures "d96" diameter of A4
  measures "d113" diameter of A5
  measures "d114" diameter of A6
  measures "d129" distance between parallel lines of L4 L2
hole "Hole4" at (-43.7683, -6.541, -32.8555) at (-27.1683, -5.453, -47.0847) at (-27.1018, -6.7323, -30.353) at (-43.2683, -9.4877, 5.6822) at (-43.681, -8.2605, -10.3677) direction (0, -0.9970894, -0.0762418) diameter 4 depth 3 counterbore diameter 4.5 counterbore depth 0.5
sketch "Sketch11" plane through (-47.2683, -15.9205, -30.8594) normal (-1, 0, 0) x (0, -0.0762418, 0.9970894)
  line L0 (-21.1011, 9.2) -> (44.1948, 9.2) projected
  line L1 (34.2694, 9.2) -> (34.2694, 0)
  line L2 (44.1948, 0) -> (-0.6602, 0) projected
  line L3 (27.1271, 9.2) -> (27.1271, 0)
  line L4 (34.2694, 9.2) -> (27.1271, 0)
  line L5 (27.1271, 9.2) -> (34.2694, 0)
  line L6 (20.1271, 9.2) -> (20.1271, 0)
  line L7 (-6.7144, 2.1) -> (-6.7144, 9.2)
  line L8 (26.1948, 9.2) -> (-21.1011, 9.2) projected
  circle A0 centre (-11.9311, 5.0192) radius 2.5
  circle A1 centre (20.1271, 3) radius 2.5
  point P0 (29.5558, 18.2269)
  point P1 (27.1271, 5.4)
  point P2 (22.6271, 5.4)
  point P3 (34.2694, 6.1999)
  point P4 (44.1948, 9.2)
  point P5 (30.6982, 4.6)
  point P6 (18.3168, 9.2)
  point P7 (14.3145, 9.2)
  point P8 (41.1296, 9.1939)
  point P9 (-21.1011, 0)
  point P10 (-21.4015, 2.0939)
  point P11 (-0.625, 2.1)
  point P12 (44.1948, 9.2)
  dimension "d98" = 5
  dimension "d115" = 5
  dimension "d116" = 0.5
  dimension "d117" = 7
  dimension "d130" = 5.2167
  constraints: 12 end point, 8 point on line, 2 centre point, 2 perpendicular, 2 vertical, 1 midpoint, 4 other
  measures "d98" diameter of A0
  measures "d115" diameter of A1
  measures "d116" distance edge to line of A1 L2
  measures "d117" distance between parallel lines of L3 L6
  measures "d130" distance from line of L7 A0.centre
hole "Hole5" at (-47.2683, -13.6743, 0.1002) at (-47.2683, -10.0062, -42.3732) at (-47.2683, -14.4637, -10.5622) direction (1, 0, 0) diameter 4 depth 3.5 counterbore diameter 4.5 counterbore depth 0.5
sketch "Sketch13" plane through (-23.6683, -19.29, 13.2067) normal (1, 0, 0) x (0, 0.0762418, -0.9970894)
  arc A0 (34.1044, -35.3) -> (29.1435, -35.3) centre (31.624, -33.2) ccw projected
  line L0 (34.1044, -35.3) -> (35.6915, -35.3) projected
  arc A1 (40.6523, -35.3) -> (35.6915, -35.3) centre (38.1719, -33.2) ccw projected
  line L1 (40.6523, -35.3) -> (47.4458, -35.3) projected
  line L2 (47.4458, -35.3) -> (47.4458, 0) projected
  line L3 (47.4458, 0) -> (40.6523, 0) projected
  arc A2 (35.6915, 0) -> (40.6523, 0) centre (38.1719, -2.1) ccw projected
  line L4 (35.6915, 0) -> (34.1044, 0) projected
  arc A3 (29.1435, 0) -> (34.1044, 0) centre (31.624, -2.1) ccw projected
  line L5 (29.1435, 0) -> (22.35, 0) projected
  line L6 (22.35, 0) -> (22.35, -35.3) projected
  line L7 (22.35, -35.3) -> (29.1435, -35.3) projected
  point P0 (14.639, 18.2269)
hole "Hole6" at (-23.6683, -18.9728, -18.4853) at (-23.6683, -18.4736, -25.0142) direction (-1, 0, 0) diameter 3.4 depth 8.8 countersink diameter 7 countersink angle 90 clearance for "Countersunk Flat Head Screw ISO 2009/7046" size "M3" standard "ISO"
chamfer "Chamfer1" distance 0.5 angle 45 2 edges at (-25.1683, -5.892, 11.1221) (-24.7091, -5.0686, 0.3536)
body "Solid2"
